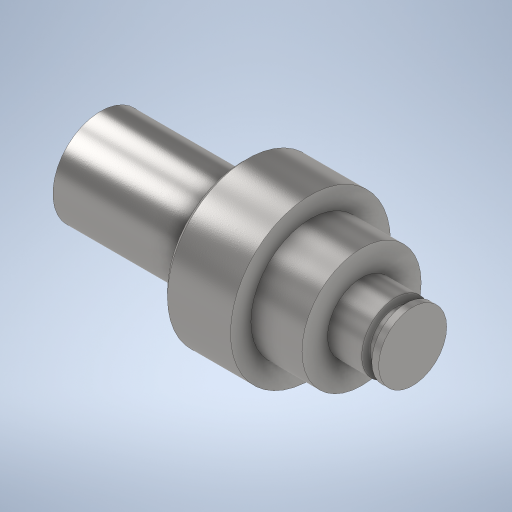
# Autodesk Inventor part: Welle
Saved by Autodesk Inventor 2024 (Build 280153000, 153)
## iProperties
Created: 2024-02-07
Part Number: Welle
Material: Stahl, galvanisiert
Document SubType Name: Modeling
Designer: ffogue
Density: 7.85 g/cm^3
Appearance: Galvanisiert
Author: ffogue
Autodesk Inventor part; units mm, degrees
ref_plane "YZ Plane" through (0, 0, 0) normal (1, 0, 0) x (0, 1, 0)
ref_plane "XZ Plane" through (0, 0, 0) normal (0, 1, 0) x (-1, 0, 0)
ref_plane "XY Plane" through (0, 0, 0) normal (0, 0, 1) x (1, 0, 0)
sketch "Skizze1" plane through (0, 0, 0) normal (0, 0, 1) x (1, 0, 0)
  line L0 (0, 0) -> (184, 0)
  line L1 (0, 0) -> (0, 28)
  line L2 (0, 28) -> (84, 28)
  line L3 (84, 28) -> (84, 47)
  line L4 (84, 47) -> (124, 47)
  line L5 (124, 47) -> (124, 35)
  line L6 (124, 35) -> (154, 35)
  line L7 (154, 35) -> (154, 20)
  line L8 (154, 20) -> (174, 20)
  line L9 (174, 20) -> (174, 15)
  line L10 (174, 15) -> (180, 15)
  line L11 (180, 15) -> (180, 20)
  line L12 (180, 20) -> (184, 20)
  line L13 (184, 20) -> (184, 0)
  dimension "d0" = 184
  dimension "d1" = 4
  dimension "d2" = 20
  dimension "d3" = 30
  dimension "d4" = 40
  dimension "d5" = 40
  dimension "d6" = 30
  dimension "d7" = 84
  dimension "d8" = 56
  dimension "d9" = 94
  dimension "d10" = 70
  constraints: 28 end point, 11 perpendicular, 2 point on line, 1 coincident, 1 horizontal, 1 vertical
  measures "d0" distance of L0.start L0.end
  measures "d1" distance between parallel lines of L13 L11
  measures "d2" distance between parallel lines of L9 L7
  measures "d3" diameter of L10 L0
  measures "d4" diameter of L12 L0
  measures "d5" distance between parallel lines of L5 L3
  measures "d6" distance between parallel lines of L7 L5
  measures "d7" distance between parallel lines of L3 L1
  measures "d8" diameter of L2 L0
  measures "d9" diameter of L4 L0
  measures "d10" diameter of L6 L0
revolve "Umdrehung1" add sketch "Skizze1" angle 360 about axis through (0, 0, 0) along (1, 0, 0)
chamfer "Fasen1" distance 4 angle 10 1 edges at (0, -28, 0) measured on face at (0, 6.9861, 6.1891)
chamfer "Fasen2" distance 3 angle 45 1 edges at (84, -47, 0)
